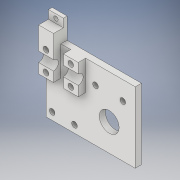
# Autodesk Inventor part: X-axis driver holder
Saved by Autodesk Inventor 2018 (Build 220112000, 112)
## iProperties
Created: 2013-10-26
Part Number: X-axis driver holder
Material: ASA Plastic
Document SubType Name: Modeling
Designer: Gabriel Smolnycki
Mass: 24.5209 g
Surface Area: 115.583 cm^2
Volume: 22.9168 cm^3
Density: 1.07 g/cm^3
Appearance: Smooth - White ASA
Sending System: SolidWorks 2017
Last Author: Gabriel Smolnycki
Last Saved: 2017-09-14
Author: Gabriel Smolnycki
Autodesk Inventor part; units mm, degrees
note: some values were not read from the file. Chosen so that the rebuilt part matches the saved one: direction of "Hole10".
ref_plane "YZ Plane" through (0, 0, 0) normal (1, 0, 0) x (0, 1, 0)
ref_plane "XZ Plane" through (0, 0, 0) normal (0, 1, 0) x (-1, 0, 0)
ref_plane "XY Plane" through (0, 0, 0) normal (0, 0, 1) x (1, 0, 0)
sketch "Sketch1" plane through (0, 0, 0) normal (0, 0, 1) x (1, 0, 0)
  line L0 (-16, 45.5) -> (-4, 45.5)
  line L1 (-16, 45.5) -> (-16, -28.5)
  line L2 (-16, -28.5) -> (56, -28.5)
  line L3 (56, 28.5) -> (-4, 28.5)
  line L4 (56, -28.5) -> (56, 28.5)
  line L5 (-4, 45.5) -> (-4, 28.5)
  constraints: 12 end point, 3 horizontal, 3 vertical
extrude "Extrusion4" add sketch "Sketch1" along normal blind 11
sketch "Sketch2" plane through (0, 0, 11) normal (0, 0, 1) x (1, 0, 0)
  line L0 (56, -28.5) -> (56, 28.5)
  line L1 (-4, 4.5) -> (-16, 4.5)
  line L2 (-4, 4.5) -> (-4, 28.5)
  line L3 (-16, 4.5) -> (-16, -28.5)
  line L4 (-16, -28.5) -> (56, -28.5)
  line L5 (56, 28.5) -> (-4, 28.5)
  constraints: 12 end point, 3 horizontal, 3 vertical
extrude "Extrusion3" cut sketch "Sketch2" against normal blind 6 draft 0
sketch "Sketch3" plane through (-4, 28.5, 0) normal (0, 1, 0) x (1, 0, 0)
  line L0 (20, -11) -> (20, -5)
  line L1 (8, -5) -> (20, -5)
  line L2 (8, -11) -> (20, -11)
  line L3 (8, -11) -> (8, -5)
  constraints: 8 end point, 2 horizontal, 2 vertical
extrude "Extrusion2" add sketch "Sketch3" against normal blind 24
sketch "Sketch4" plane through (-16, 45.5, 0) normal (0, 1, 0) x (1, 0, 0)
  line L0 (12, -11) -> (0, -11)
  line L1 (0, -11) -> (0, -3)
  line L2 (12, -11) -> (12, -3)
  line L3 (12, -3) -> (0, -3)
  constraints: 8 end point, 2 horizontal, 2 vertical
extrude "Extrusion1" cut sketch "Sketch4" against normal blind 6.75
hole "Hole10" at (-10, 42.25, 3) direction (0, 0, -1) diameter 3.5 depth 3
hole "Hole9" at (24, 13.5, 0) direction (0, 0, 1) diameter 4.5 depth 5
hole "Hole8" at (46, 13.5, 0) direction (0, 0, 1) diameter 4.5 depth 5
hole "Hole7" at (7, -22.5, 0) direction (0, 0, 1) diameter 4.5 depth 5
hole "Hole6" at (-11, -22.5, 0) direction (0, 0, 1) diameter 4.5 depth 5
sketch "Sketch9" plane through (0, 0, 0) normal (0, 0, 1) x (1, 0, 0)
  point P0 (-11, -22.5)
hole "Hole5" at (35, -6.5, 0) direction (0, 0, 1) diameter 16 depth 5
sketch "Sketch8" plane through (0, 0, 0) normal (0, 0, 1) x (1, 0, 0)
  point P0 (7, -22.5)
hole "Hole4" at (10, 8.5, 0) direction (0, 0, 1) diameter 4.5 depth 11
sketch "Sketch7" plane through (0, 0, 0) normal (0, 0, 1) x (1, 0, 0)
  point P0 (46, 13.5)
hole "Hole3" at (10, 24.5, 0) direction (0, 0, 1) diameter 4.5 depth 11
sketch "Sketch6" plane through (0, 0, 0) normal (0, 0, 1) x (1, 0, 0)
  point P0 (24, 13.5)
hole "Hole2" at (-10, 8.5, 0) direction (0, 0, 1) diameter 4.5 depth 11
sketch "Sketch5" plane through (-16, 45.5, 3) normal (0, 0, 1) x (1, 0, 0)
  point P0 (6, -3.25)
hole "Hole1" at (-10, 24.5, 0) direction (0, 0, 1) diameter 4.5 depth 11
sketch "Sketch15" plane through (0, 0, 11) normal (0, 0, 1) x (1, 0, 0)
  line L0 (4, 20.5) -> (16, 20.5)
  line L1 (4, 20.5) -> (4, 16.5)
  line L2 (16, 20.5) -> (16, 16.5)
  line L3 (4, 16.5) -> (16, 16.5)
  line L4 (4, 16.5) -> (14, 16.5)
  constraints: 10 end point, 3 horizontal, 2 vertical
revolve "Revolution2" cut sketch "Sketch15" angle 180 about axis through (4, 16.5, 11) along (-1, 0, 0)
sketch "Sketch16" plane through (4, 28.5, 11) normal (0, 0, 1) x (1, 0, 0)
  line L0 (-8, -8) -> (-20, -8)
  line L1 (-8, -8) -> (-8, -12)
  line L2 (-20, -8) -> (-20, -12)
  line L3 (-8, -12) -> (-20, -12)
  line L4 (-8, -12) -> (-18, -12)
  constraints: 10 end point, 3 horizontal, 2 vertical
revolve "Revolution1" cut sketch "Sketch16" angle 180 about axis through (-4, 16.5, 11) along (-1, 0, 0)
sketch "Sketch10" plane through (0, 0, 0) normal (0, 0, 1) x (1, 0, 0)
  point P0 (35, -6.5)
sketch "Sketch11" plane through (0, 0, 0) normal (0, 0, 1) x (1, 0, 0)
  point P0 (10, 8.5)
sketch "Sketch12" plane through (0, 0, 0) normal (0, 0, 1) x (1, 0, 0)
  point P0 (10, 24.5)
sketch "Sketch13" plane through (0, 0, 0) normal (0, 0, 1) x (1, 0, 0)
  point P0 (-10, 8.5)
sketch "Sketch14" plane through (0, 0, 0) normal (0, 0, 1) x (1, 0, 0)
  point P0 (-10, 24.5)
body "Solid3"
